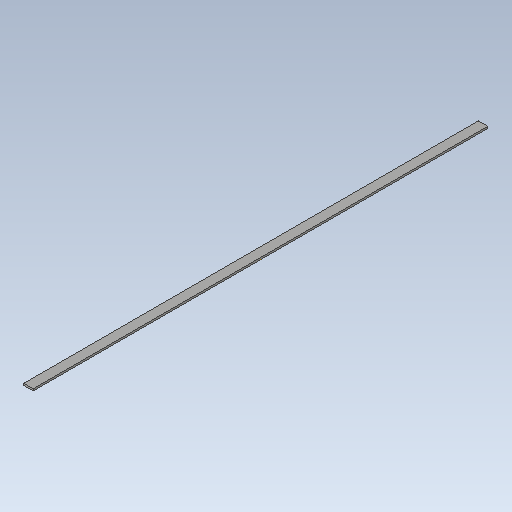
# Autodesk Inventor part: håndfang
Saved by Autodesk Inventor 2020.1 (Build 241239000, 239)
## iProperties
Created: 2019-09-28
Part Number: håndfang
Material: S235JR
Document SubType Name: Modeling
Designer: loppen
Density: 7.85 g/cm^3
Appearance: Light Gray
Mass: 1186.28 g
Surface Area: 727.87 cm^2
Volume: 151.119 cm^3
Author: loppen
Autodesk Inventor part; units mm, degrees
ref_plane "YZ Plane" through (0, 0, 0) normal (1, 0, 0) x (0, 1, 0)
ref_plane "XZ Plane" through (0, 0, 0) normal (0, 1, 0) x (-1, 0, 0)
ref_plane "XY Plane" through (0, 0, 0) normal (0, 0, 1) x (1, 0, 0)
sketch "Sketch1" plane through (0, 0, 0) normal (0, 0, 1) x (1, 0, 0)
  line L0 (0, 0) -> (25, 0)
  line L1 (25, 0) -> (25, 5)
  line L2 (25, 5) -> (0, 5)
  line L3 (0, 5) -> (0, 0)
  dimension "d0" = 25
  dimension "d1" = 5
  constraints: 8 end point, 2 parallel, 1 horizontal, 1 perpendicular
  measures "d0" distance of L0.start L0.end
  measures "d1" distance of L0.end L1.end
extrude "Extrusion1" add sketch "Sketch1" along normal mid plane 1208.95
body "Solid1"
